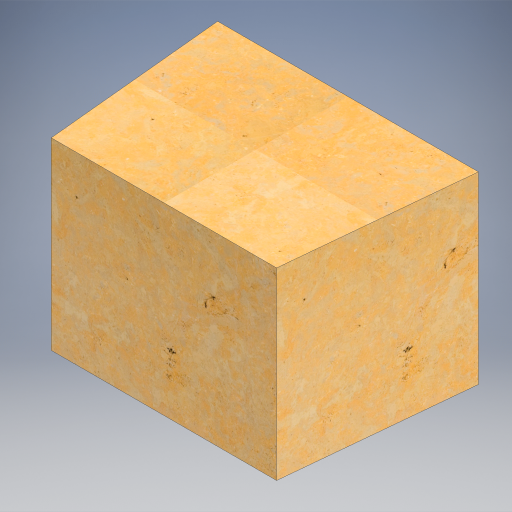
# Autodesk Inventor part: Boulder wall block - 20
Saved by Autodesk Inventor 2023 (Build 270158030, 158C)
## iProperties
RuleStatus: InUse
Created: 2022-05-23
Part Number: Boulder wall block - 20
Material: Granite, Cut, Polished
Document SubType Name: Modeling
Designer: awelt
Mass: 807601 g
Surface Area: 27093.4 cm^2
Volume: 299111 cm^3
Density: 2.7 g/cm^3
Appearance: Amber Select
AfterDocSave0: Convert in3 volume to ft3
in3 to ft3: 0.01
TEST: 0.006
Author: awelt
Autodesk Inventor part; units mm, degrees
ref_plane "YZ Plane" through (0, 0, 0) normal (1, 0, 0) x (0, 1, 0)
ref_plane "XZ Plane" through (0, 0, 0) normal (0, 1, 0) x (-1, 0, 0)
ref_plane "XY Plane" through (0, 0, 0) normal (0, 0, 1) x (1, 0, 0)
sketch "Sketch1" plane through (0, 0, 0) normal (0, 1, 0) x (-1, 0, 0)
  line L0 (-58.6978, 0) -> (-804.9022, 0)
  line L1 (-863.6, 0) -> (-863.6, -609.6) construction
  line L2 (-863.6, -609.6) -> (0, -609.6)
  line L3 (0, -609.6) -> (0, 0) construction
  line L4 (0, -609.6) -> (-58.6978, 0)
  line L5 (-863.6, -609.6) -> (-804.9022, 0)
  line L6 (-431.8, -609.6) -> (-431.8, 0) construction
  dimension "d0" = 863.6
  dimension "d1" = 609.6
  dimension "d2" = 11
  dimension "d5" = 609.6
  constraints: 14 end point, 2 midpoint, 2 parallel, 1 horizontal, 1 perpendicular, 1 other
  measures "d0" distance of L2.end L1.end
  measures "d1" distance of L1.end L1.start
  measures "d2" angle of L4 L5
  measures "d5" distance between parallel lines of L2 L0
extrude "Extrusion1" add sketch "Sketch1" along normal blind 609.6
equation "\"d5\" = d1"
body "Solid1"
